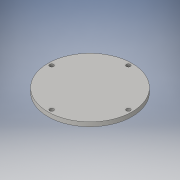
# Autodesk Inventor part: Acrylic Lens
Saved by Autodesk Inventor 2016 (Build 200138000, 138)
## iProperties
Created: 2017-09-28
Part Number: Acrylic Lens
Material: Generic
Document SubType Name: Modeling
Designer: Student
Density: 1 g/cm^3
Appearance: Default
Author: Student
Autodesk Inventor part; units mm, degrees
ref_plane "YZ Plane" through (0, 0, 0) normal (1, 0, 0) x (0, 1, 0)
ref_plane "XZ Plane" through (0, 0, 0) normal (0, 1, 0) x (-1, 0, 0)
ref_plane "XY Plane" through (0, 0, 0) normal (0, 0, 1) x (1, 0, 0)
sketch "Sketch1" plane through (0, 0, 0) normal (0, 1, 0) x (-1, 0, 0)
  circle A0 centre (0, 0) radius 31.75
  dimension "d0" = 63.5
  constraints: 1 centre point, 1 coincident
  measures "d0" diameter of A0
extrude "Extrusion1" add sketch "Sketch1" along normal blind 3.175
sketch "Sketch2" plane through (0, 0, 0) normal (0, -1, 0) x (1, 0, 0)
  point P0 (0, 0)
  point P1 (-28.956, 0)
  point P2 (0, -28.956)
  point P3 (28.956, 0)
  point P4 (0, 28.956)
  dimension "d3" = 28.956
  dimension "d6" = 360
  constraints: 5 other
  measures "d3" distance of point (0, 0) point (-28.956, 0)
hole "Hole1" at (-28.956, 0, 0) at (0, 0, 28.956) at (28.956, 0, 0) at (0, 0, -28.956) direction (0, 1, 0) diameter 3 depth 25.4 tip angle 118
body "Solid1"
